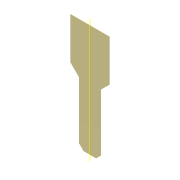
# Autodesk Inventor part: 32ch_ECoG
Saved by Autodesk Inventor 2014 (Build 180170000, 170)
## iProperties
Created: 2016-08-28
Part Number: 32ch_ECoG
Material: Generic
Document SubType Name: Modeling
Designer: Camilo
Density: 1 g/cm^3
Appearance: Clear - Amber
Author: Camilo
Autodesk Inventor part; units mm, degrees
ref_plane "YZ Plane" through (0, 0, 0) normal (1, 0, 0) x (0, 1, 0)
ref_plane "XZ Plane" through (0, 0, 0) normal (0, 1, 0) x (-1, 0, 0)
ref_plane "XY Plane" through (0, 0, 0) normal (0, 0, 1) x (1, 0, 0)
sketch "Sketch1" plane through (0, 0, 0) normal (0, 1, 0) x (-1, 0, 0)
  line L0 (6.4687, 18.4347) -> (6.4687, 11.6025)
  line L1 (6.4687, 11.6025) -> (5.0549, 10.1887)
  line L2 (5.0549, 10.1887) -> (5.0549, 0.787)
  line L3 (5.0549, 0.787) -> (4.2803, 0.0124)
  line L4 (4.2803, 0.0124) -> (2.207, 0.0124)
  line L5 (2.207, 0.0124) -> (1.4324, 0.787)
  line L6 (1.4324, 0.787) -> (1.4324, 10.1729)
  line L7 (1.4324, 10.1729) -> (1.4324, 10.1887)
  line L8 (1.4324, 10.1887) -> (0.0187, 11.6025)
  line L9 (0.0187, 11.6025) -> (0.0187, 18.4347)
  line L10 (0.0187, 18.4347) -> (6.4687, 18.4347)
  point P0 (0, 0)
  constraints: 22 end point
extrude "Extrusion1" add sketch "Sketch1" along normal blind 0.05
ref_plane "Work Plane1" through (-3.2437, 0, 18.4347) normal (1, 0, 0) x (0, 0, -1)
body "Solid1"
